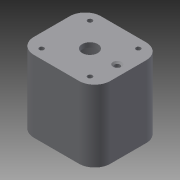
# Autodesk Inventor part: Drill-NEMA17_Adapter
Saved by Autodesk Inventor 2015 (Build 190159000, 159)
## iProperties
Created: 2015-10-01
Part Number: Drill-NEMA17_Adapter
Material: Generic
Document SubType Name: Modeling
Designer: Kurtis
Density: 1 g/cm^3
Appearance: Default
Author: Kurtis
Autodesk Inventor part; units mm, degrees
ref_plane "YZ Plane" through (0, 0, 0) normal (1, 0, 0) x (0, 1, 0)
ref_plane "XZ Plane" through (0, 0, 0) normal (0, 1, 0) x (-1, 0, 0)
ref_plane "XY Plane" through (0, 0, 0) normal (0, 0, 1) x (1, 0, 0)
sketch "Sketch1" plane through (0, 0, 0) normal (0, 0, 1) x (1, 0, 0)
  line L0 (0, 0) -> (0, 39)
  line L1 (0, 39) -> (45, 39)
  line L2 (45, 39) -> (45, 0)
  line L3 (45, 0) -> (0, 0)
  line L4 (0, 39) -> (-2, 39) construction
  line L5 (-2, 39) -> (-2, 41) construction
  line L6 (-2, 41) -> (47, 41)
  line L7 (47, 41) -> (47, -2)
  line L8 (47, -2) -> (-2, -2)
  line L9 (-2, -2) -> (-2, 41)
  dimension "d0" = 39
  dimension "d1" = 45
  dimension "d2" = 2
  dimension "d3" = 2
  dimension "d4" = 49
  dimension "d5" = 43
  dimension "d6" = 49
  constraints: 20 end point, 7 perpendicular, 1 point on line, 1 vertical
  measures "d0" distance of L0.start L0.end
  measures "d1" distance of L0.end L1.end
  measures "d2" distance of L0.end L4.end
  measures "d3" distance of L4.end L5.end
  measures "d4" distance of L5.end L6.end
  measures "d5" distance of L6.end L7.end
  measures "d6" distance of L7.end L8.end
extrude "Extrusion1" add sketch "Sketch1" along normal blind 43
sketch "Sketch2" plane through (0, 0, 43) normal (0, 0, 1) x (1, 0, 0)
  line L0 (-2, -2) -> (47, 41) construction
  line L1 (47, 41) -> (-2, 41)
  line L2 (47, 41) -> (-2, 41) projected
  line L3 (-2, 41) -> (22.5, 19.5) construction
  line L4 (-2, 41) -> (-2, -2)
  line L5 (-2, -2) -> (47, -2)
  line L6 (-2, -2) -> (47, -2) projected
  line L7 (47, -2) -> (47, 41)
  line L8 (-2, 41) -> (47, 41)
  circle A0 centre (22.5, 19.5) radius 5
  line L9 (27.5, 19.5) -> (40, 19.5) construction
  circle A1 centre (40, 19.5) radius 1.75
  point P0 (0, 0)
  dimension "d9" = 10
  dimension "d12" = 12.5
  dimension "d13" = 3.5
  dimension "d14" = 21.5
  constraints: 16 end point, 2 coincident, 2 collinear, 2 perpendicular, 1 centre point, 1 horizontal, 1 horizontal alignment, 1 midpoint, 2 other
  measures "d12" distance of L9.start L9.end
  measures "d13" diameter of A1
  measures "d14" distance between parallel lines of L6 L9
extrude "Extrusion3" add sketch "Sketch2" along normal blind 3
fillet "Fillet1" radius 10 8 edges at (-2, 41, 23) (0, 39, 21.5) (0, 0, 21.5) (-2, -2, 23) (47, -2, 23) (45, 0, 21.5) (47, 41, 23) (45, 39, 21.5)
chamfer "Chamfer1" distance 1 angle 45 1 edges at (38.25, 19.5, 46)
sketch "Sketch3" plane through (0, 0, 46) normal (0, 0, 1) x (1, 0, 0)
  circle A0 centre (22.5, 19.5) radius 5 construction
  line L0 (22.5, 19.5) -> (22.5, 41) construction
  line L1 (37, 41) -> (8, 41) construction
  line L2 (22.5, 19.5) -> (22.5, -2) construction
  line L3 (8, -2) -> (37, -2) construction
  line L4 (22.5, 19.5) -> (47, 19.5) construction
  line L5 (47, 19.5) -> (22.5, 19.5) construction
  line L6 (-2.181, 19.5) -> (22.5, 19.5) construction
  line L7 (38, 35) -> (38, 4) construction
  line L8 (38, 4) -> (7, 4) construction
  line L9 (7, 4) -> (7, 35) construction
  line L10 (7, 35) -> (38, 35) construction
  line L11 (38, 35) -> (7, 4) construction
  line L12 (38, 4) -> (7, 35) construction
  circle A1 centre (38, 35) radius 1.5
  circle A2 centre (7, 35) radius 1.5
  circle A3 centre (7, 4) radius 1.5
  circle A4 centre (38, 4) radius 1.5
  point P0 (0, 0)
  dimension "d22" = 31
  dimension "d23" = 31
  dimension "d24" = 3
  dimension "d25" = 3
  dimension "d26" = 3
  dimension "d27" = 3
  constraints: 22 end point, 4 centre point, 4 coincident, 4 midpoint, 2 collinear, 2 parallel, 1 horizontal, 1 perpendicular, 1 point on line
  measures "d22" distance of L7.start L7.end
  measures "d23" distance of L7.end L8.end
  measures "d24" diameter of A1
  measures "d25" diameter of A2
  measures "d26" diameter of A3
  measures "d27" diameter of A4
extrude "Extrusion4" cut sketch "Sketch3" against normal blind 57.5
body "Solid1"
